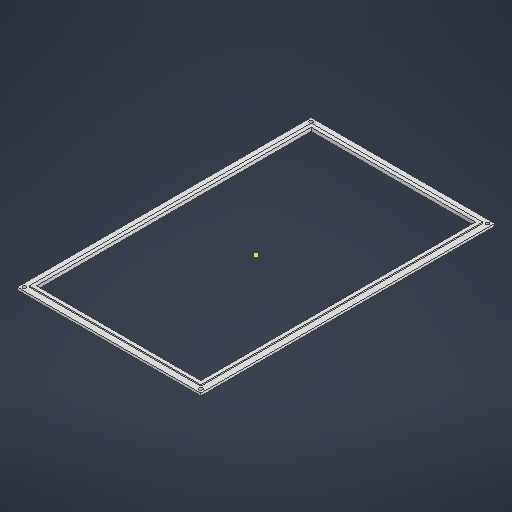
# Autodesk Inventor part: LCD_Bottom_Cover
Saved by Autodesk Inventor 2026.2 (Build 302298010, 298A)
## iProperties
Created: 2026-08-14
Part Number: LCD_Bottom_Cover
Material: 일반
Document SubType Name: Modeling
Designer: User
Density: 1 g/cm^3
Appearance: 기본값
Author: User
Autodesk Inventor part; units mm, degrees
ref_plane "YZ Plane" through (0, 0, 0) normal (1, 0, 0) x (0, 1, 0)
ref_plane "XZ Plane" through (0, 0, 0) normal (0, 1, 0) x (-1, 0, 0)
ref_plane "XY Plane" through (0, 0, 0) normal (0, 0, 1) x (1, 0, 0)
sketch "스케치1" plane through (0, 0, 0) normal (0, 1, 0) x (-1, 0, 0)
  line L0 (76.5, 122.5) -> (-76.5, 122.5)
  line L1 (-76.5, 122.5) -> (-76.5, -122.5)
  line L2 (-76.5, -122.5) -> (76.5, -122.5)
  line L3 (76.5, -122.5) -> (76.5, 122.5)
  line L4 (76.5, 122.5) -> (-76.5, -122.5) construction
  line L5 (-76.5, 122.5) -> (76.5, -122.5) construction
  line L6 (68.5, 114.5) -> (-68.5, 114.5)
  line L7 (-68.5, 114.5) -> (-68.5, -114.5)
  line L8 (-68.5, -114.5) -> (68.5, -114.5)
  line L9 (68.5, -114.5) -> (68.5, 114.5)
  line L10 (73.5, 119.5) -> (-73.5, 119.5) construction
  line L11 (-73.5, 119.5) -> (-73.5, -119.5) construction
  line L12 (-73.5, -119.5) -> (73.5, -119.5) construction
  line L13 (73.5, -119.5) -> (73.5, 119.5) construction
  circle A0 centre (73.5, 119.5) radius 1.5
  line L14 (0, 146) -> (0, -170.2735) construction
  line L15 (-97, 0) -> (111, 0) construction
  circle A1 centre (-73.5, 119.5) radius 1.5
  circle A2 centre (73.5, -119.5) radius 1.5
  circle A3 centre (-73.5, -119.5) radius 1.5
  point P0 (0, 0)
  dimension "d0" = 245
  dimension "d1" = 153
  dimension "d2" = 8
  dimension "d3" = 3
  dimension "d4" = 3
  constraints: 32 end point, 6 parallel, 4 centre point, 4 perpendicular, 3 symmetric about line, 2 midpoint, 1 coincident, 1 horizontal, 1 point on line, 1 vertical, 9 other
  measures "d0" distance of L2.end L0.start
  measures "d1" distance of L1.end L2.end
  measures "d2" distance between parallel lines of L3 L9
  measures "d3" distance between parallel lines of L3 L13
  measures "d4" diameter of A0
extrude "돌출1" add sketch "스케치1" along normal blind 2
sketch "스케치2" plane through (0, 2, 0) normal (0, 1, 0) x (1, 0, 0)
  point P0 (0, 0)
sketch "스케치3" plane through (0, 2, 0) normal (0, 1, 0) x (1, 0, 0)
  line L0 (-76.5, -122.5) -> (76.5, -122.5) projected
  line L1 (-76.5, 122.5) -> (-76.5, -122.5) projected
  line L2 (76.5, 122.5) -> (-76.5, 122.5) projected
  line L3 (76.5, -122.5) -> (76.5, 122.5) projected
  line L4 (71.5, -117.5) -> (-71.5, -117.5)
  line L5 (-71.5, -117.5) -> (-71.5, 117.5)
  line L6 (-71.5, 117.5) -> (71.5, 117.5)
  line L7 (71.5, 117.5) -> (71.5, -117.5)
  line L8 (68.5, -114.5) -> (-68.5, -114.5) projected
  line L9 (-68.5, -114.5) -> (-68.5, 114.5) projected
  line L10 (-68.5, 114.5) -> (68.5, 114.5) projected
  line L11 (68.5, 114.5) -> (68.5, -114.5) projected
  line L12 (-68.5, -114.5) -> (68.5, -114.5)
  line L13 (68.5, -114.5) -> (68.5, 114.5)
  line L14 (68.5, 114.5) -> (-68.5, 114.5)
  line L15 (-68.5, 114.5) -> (-68.5, -114.5)
  point P0 (0, 0)
  dimension "d7" = 5
  constraints: 16 end point, 2 parallel, 1 horizontal, 1 perpendicular, 3 other
  measures "d7" distance between parallel lines of L0 L4
extrude "돌출2" add sketch "스케치3" along normal blind 1 contours L4 L5 L6 L7
